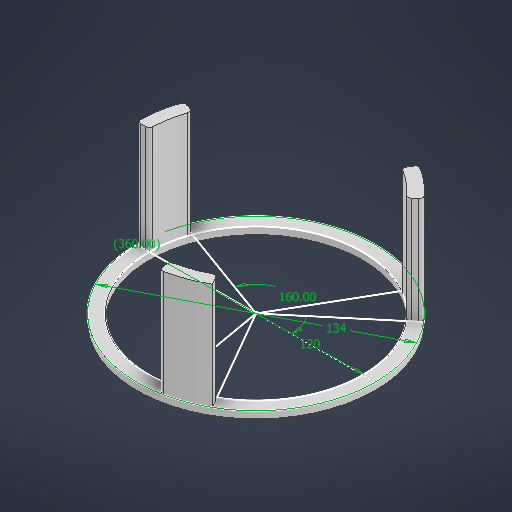
# Autodesk Inventor part: Stand
Saved by Autodesk Inventor 2026.2 (Build 302298000, 298)
## iProperties
Created: 2026-01-26
Part Number: Stand
Material: Generic
Document SubType Name: Modeling
Designer: Cobble
Density: 1 g/cm^3
Appearance: Default
Author: Cobble
Autodesk Inventor part; units mm, degrees
ref_plane "YZ Plane" through (0, 0, 0) normal (1, 0, 0) x (0, 1, 0)
ref_plane "XZ Plane" through (0, 0, 0) normal (0, 1, 0) x (-1, 0, 0)
ref_plane "XY Plane" through (0, 0, 0) normal (0, 0, 1) x (1, 0, 0)
sketch "Sketch1" plane through (0, 0, 0) normal (0, 0, 1) x (1, 0, 0)
  circle A0 centre (0, 0) radius 67
  circle A1 centre (0, 0) radius 60
  line L0 (0, 0) -> (-67, 0)
  line L1 (0, 0) -> (-62.9594, 22.9153)
  line L2 (0, 0) -> (67, 0) construction
  line L3 (0, 0) -> (33.5, -58.0237)
  line L4 (0, 0) -> (11.6344, -65.9821)
  line L5 (0, 0) -> (33.5, 58.0237)
  line L6 (0, 0) -> (51.325, 43.0668)
  point P0 (10.4189, -59.0885)
  point P1 (30, -51.9615)
  point P2 (45.9627, 38.5673)
  point P3 (30, 51.9615)
  point P4 (-56.3816, 20.5212)
  point P5 (-60, 0)
  dimension "d0" = 134
  dimension "d1" = 120
  dimension "d2" = 160
  dimension "d5" = 360
  constraints: 14 end point, 4 coincident, 2 centre point, 2 horizontal, 2 point on circle, 1 equal length, 17 other
  measures "d0" diameter of A0
  measures "d1" diameter of A1
  measures "d2" angle of L2 L1
extrude "Extrusion1" add sketch "Sketch1" against normal blind 4 contours A0 L3 A1 L6 | L6 A1 L5 A0 | A0 L4 A1 L3 | L5 A1 L1 A0 | A0 L0 A1 L4 | L1 A1 L0 A0
extrude "Extrusion2" add sketch "Sketch1" along normal blind 60 contours L6 A1 L5 A0 | A0 L4 A1 L3 | L1 A1 L0 A0
fillet "Fillet1" radius 2 11 edges at (-62.9594, 22.9153, 30) (-67, 0, 30) (-56.3816, 20.5212, 30) (-60, 0, 30) (33.5, 58.0237, 30) (51.325, 43.0668, 30) (45.9627, 38.5673, 30) (30, 51.9615, 30) (11.6344, -65.9821, 30) (10.4189, -59.0885, 30) (30, -51.9615, 30)
body "Solid1"
